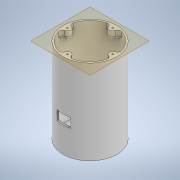
# Autodesk Inventor part: Wrist
Saved by Autodesk Inventor 2021 (Build 250183000, 183)
## iProperties
Created: 2022-07-05
Part Number: Wrist
Material: Ogólny
Document SubType Name: Modeling
Designer: MicnedSQ
Density: 1 g/cm^3
Appearance: Domyślna
Author: MicnedSQ
Autodesk Inventor part; units mm, degrees
ref_plane "YZ Plane" through (0, 0, 0) normal (1, 0, 0) x (0, 1, 0)
ref_plane "XZ Plane" through (0, 0, 0) normal (0, 1, 0) x (-1, 0, 0)
ref_plane "XY Plane" through (0, 0, 0) normal (0, 0, 1) x (1, 0, 0)
sketch "Szkic1" plane through (0, 0, 0) normal (0, 1, 0) x (-1, 0, 0)
  circle A0 centre (0, 0) radius 31.8198
  line L0 (-21.15, 21.15) -> (21.15, 21.15)
  line L1 (21.15, 21.15) -> (21.15, -21.15)
  line L2 (21.15, -21.15) -> (-21.15, -21.15)
  line L3 (-21.15, -21.15) -> (-21.15, 21.15)
  line L4 (-21.15, 21.15) -> (21.15, -21.15) construction
  line L5 (21.15, 21.15) -> (-21.15, -21.15) construction
  dimension "d2" = 42.3
  dimension "d3" = 42.3
  constraints: 12 end point, 2 midpoint, 2 parallel, 1 centre point, 1 coincident, 1 horizontal, 1 perpendicular
  measures "d2" distance of L1.end L2.end
  measures "d3" distance of L0.end L1.end
extrude "Wyciągnięcie proste1" add sketch "Szkic1" along normal blind 100 contours A0 | L0 L1 L2 L3
shell "Skorupa1" thickness 2 removed faces 1 at (6.1204, 100, 14.4125)
sketch "Szkic2" plane through (0, 2, 0) normal (0, 1, 0) x (1, 0, 0)
  line L0 (-21.15, -21.15) -> (21.15, -21.15)
  line L1 (21.15, -21.15) -> (21.15, 21.15)
  line L2 (21.15, 21.15) -> (-21.15, 21.15)
  line L3 (-21.15, 21.15) -> (-21.15, -21.15)
  line L4 (-21.15, -21.15) -> (21.15, 21.15) construction
  line L5 (21.15, -21.15) -> (-21.15, 21.15) construction
  point P0 (0, 0)
  point P1 (-15.51, 15.51)
  point P2 (-15.51, -15.51)
  point P3 (15.51, 15.51)
  point P4 (15.51, -15.51)
  dimension "d7" = 42.3
  dimension "d8" = 42.3
  dimension "d16" = 5.64
  dimension "d19" = 31.02
  dimension "d22" = 31.02
  constraints: 12 end point, 2 horizontal, 2 midpoint, 2 parallel, 1 perpendicular, 1 point on line, 1 vertical, 3 other
  measures "d7" distance of L2.end L1.end
  measures "d8" distance of L1.end L0.end
  measures "d16" distance from line of point (-15.51, 15.51) L2
  measures "d19" distance of point (-15.51, 15.51) point (-15.51, -15.51)
  measures "d22" distance of point (-15.51, 15.51) point (15.51, 15.51)
hole "Otwór1" at (0, 2, 0) direction (0, -1, 0) diameter 22 end through all
hole "Otwór2" at (-15.51, 2, -15.51) at (-15.51, 2, 15.51) at (15.51, 2, -15.51) at (15.51, 2, 15.51) direction (0, -1, 0) diameter 3 end through all
ref_plane "Płaszczyzna konstrukcyjna1" through (-21.15, 2, 21.15) normal (0, 0, 1) x (1, 0, 0)
sketch "Szkic3" plane through (-21.15, 2, 21.15) normal (0, 0, 1) x (1, 0, 0)
  line L0 (13.15, 28.3) -> (29.15, 28.3)
  line L1 (29.15, 28.3) -> (29.15, 39.3)
  line L2 (29.15, 39.3) -> (13.15, 39.3)
  line L3 (13.15, 39.3) -> (13.15, 28.3)
  line L4 (13.15, 28.3) -> (29.15, 39.3) construction
  line L5 (29.15, 28.3) -> (13.15, 39.3) construction
  line L6 (52.9698, -2) -> (-10.6698, -2) projected
  point P0 (21.15, -2)
  point P1 (21.15, 33.8)
  dimension "d33" = 16
  dimension "d34" = 11
  dimension "d35" = 41.3
  constraints: 12 end point, 2 midpoint, 2 parallel, 1 horizontal, 1 perpendicular
  measures "d33" distance of L2.end L1.end
  measures "d34" distance of L1.end L0.end
  measures "d35" distance between parallel lines of L6 L2
extrude "Wyciągnięcie proste2" cut sketch "Szkic3" along normal blind 15
ref_plane "Płaszczyzna konstrukcyjna2" through (0, 100, 0) normal (0, 1, 0) x (1, 0, 0)
sketch "Szkic5" plane through (0, 100, 0) normal (0, 1, 0) x (1, 0, 0)
  circle A0 centre (0, 26.82) radius 4
  circle A1 centre (-26.82, 0) radius 4
  circle A2 centre (0, -26.82) radius 4
  circle A3 centre (26.82, 0) radius 4
  point P0 (0, 0)
  dimension "d39" = 8
  dimension "d40" = 26.82
  dimension "d43" = 360
  constraints: 4 centre point, 9 other
  measures "d39" diameter of A0
  measures "d40" distance of A0.centre point (0, 0)
extrude "Wyciągnięcie proste3" add sketch "Szkic5" against normal blind 10
fillet "Zaokrąglenie1" radius 4 12 edges at (-2.787, 95, -29.6893) (2.787, 95, -29.6893) (29.6893, 95, 2.787) (-29.6893, 95, 2.787) (-2.787, 95, 29.6893) (29.6893, 95, -2.787) (2.787, 95, 29.6893) (-29.6893, 95, -2.787) (22.82, 90, 0) (0, 90, -22.82) (0, 90, 22.82) (-22.82, 90, 0)
sketch "Szkic6" plane through (0, 100, 0) normal (0, 1, 0) x (1, 0, 0)
  arc A0 (-25.7327, -3.8494) -> (-25.7327, 3.8494) centre (-26.82, 0) ccw projected
  point P0 (0, 0)
  point P1 (-26.82, 0)
  dimension "d48" = 0
  measures "d48" distance of A0.centre point (-26.82, 0)
hole "Otwór3" at (-26.82, 100, 0) direction (0, -1, 0) diameter 1.778 depth 6 tip angle 118
pattern_circular "Szyk kołowy1" count 4 over 360 about axis through (0, 0, 0) along (0, 1, 0) of "Otwór3"
